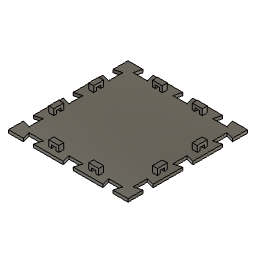
5 Power_source2 v14 (Autodesk Fusion 360 archive; units mm, degrees)
design "0 base_tile"
Autodesk Fusion 360 part; units mm, degrees
sketch "Sketch1" plane through (0, 0, 0) normal (0, 0, 1) x (1, 0, 0)
  line L0 (60, 60) -> (-60, 60)
  line L1 (-60, 60) -> (-60, -60)
  line L2 (-60, -60) -> (60, -60)
  line L3 (60, -60) -> (60, 60)
  line L4 (60, 60) -> (-60, -60) construction
  line L5 (-60, 60) -> (60, -60) construction
  dimension "d78" = 120
  dimension "d79" = 120
  constraint horizontal L0
  constraint perpendicular L0 L1
  constraint parallel L0 L2
  constraint parallel L1 L3
  constraint coincident L4 origin
  constraint coincident L5 origin
  measures "d78" distance of L1.end L2.end
  measures "d79" distance of L0.end L1.end
extrude "Extrude1" add sketch "Sketch1" along normal blind 3 makes body 1
sketch "Sketch3" plane through (0, 0, 3) normal (0, 0, 1) x (-1, 0, 0)
  line L0 (-60, 60) -> (-60, -60)
  line L1 (-60, -60) -> (60, -60)
  line L2 (60, -60) -> (60, 60)
  line L3 (60, 60) -> (-60, 60)
  line L4 (0, 60) -> (-5, 60)
  line L5 (0, 60) -> (5, 60)
  line L6 (5, 60) -> (7.0706, 52.2726)
  line L7 (5, 60) -> (13, 60) construction
  line L8 (-5, 60) -> (-7.0706, 52.2726)
  line L9 (-5, 60) -> (3, 60) construction
  line L10 (-7.0706, 52.2726) -> (7.0706, 52.2726)
  line L11 (-35, 60) -> (-32.9294, 52.2726)
  line L12 (-40, 60) -> (-35, 60)
  line L13 (-40, 60) -> (-45, 60)
  line L14 (-45, 60) -> (-47.0706, 52.2726)
  line L15 (-47.0706, 52.2726) -> (-32.9294, 52.2726)
  line L16 (45, 60) -> (47.0706, 52.2726)
  line L17 (40, 60) -> (45, 60)
  line L18 (40, 60) -> (35, 60)
  line L19 (35, 60) -> (32.9294, 52.2726)
  line L20 (32.9294, 52.2726) -> (47.0706, 52.2726)
  line L21 (-60, 45) -> (-52.2726, 47.0706)
  line L22 (-60, 40) -> (-60, 45)
  line L23 (-60, 40) -> (-60, 35)
  line L24 (-52.2726, 32.9294) -> (-52.2726, 47.0706)
  line L25 (-60, 35) -> (-52.2726, 32.9294)
  line L26 (-60, 5) -> (-52.2726, 7.0706)
  line L27 (-60, 0) -> (-60, 5)
  line L28 (-60, 0) -> (-60, -5)
  line L29 (-60, -5) -> (-52.2726, -7.0706)
  line L30 (-52.2726, -7.0706) -> (-52.2726, 7.0706)
  line L31 (-60, -35) -> (-52.2726, -32.9294)
  line L32 (-60, -40) -> (-60, -35)
  line L33 (-60, -40) -> (-60, -45)
  line L34 (-60, -45) -> (-52.2726, -47.0706)
  line L35 (-52.2726, -47.0706) -> (-52.2726, -32.9294)
  line L36 (-45, -60) -> (-47.0706, -52.2726)
  line L37 (-40, -60) -> (-45, -60)
  line L38 (-40, -60) -> (-35, -60)
  line L39 (-32.9294, -52.2726) -> (-47.0706, -52.2726)
  line L40 (-35, -60) -> (-32.9294, -52.2726)
  line L41 (-5, -60) -> (-7.0706, -52.2726)
  line L42 (0, -60) -> (-5, -60)
  line L43 (0, -60) -> (5, -60)
  line L44 (5, -60) -> (7.0706, -52.2726)
  line L45 (7.0706, -52.2726) -> (-7.0706, -52.2726)
  line L46 (35, -60) -> (32.9294, -52.2726)
  line L47 (40, -60) -> (35, -60)
  line L48 (40, -60) -> (45, -60)
  line L49 (45, -60) -> (47.0706, -52.2726)
  line L50 (47.0706, -52.2726) -> (32.9294, -52.2726)
  line L51 (60, -45) -> (52.2726, -47.0706)
  line L52 (60, -40) -> (60, -45)
  line L53 (60, -40) -> (60, -35)
  line L54 (52.2726, -32.9294) -> (52.2726, -47.0706)
  line L55 (60, -35) -> (52.2726, -32.9294)
  line L56 (60, -5) -> (52.2726, -7.0706)
  line L57 (60, 0) -> (60, -5)
  line L58 (60, 0) -> (60, 5)
  line L59 (60, 5) -> (52.2726, 7.0706)
  line L60 (52.2726, 7.0706) -> (52.2726, -7.0706)
  line L61 (60, 35) -> (52.2726, 32.9294)
  line L62 (60, 40) -> (60, 35)
  line L63 (60, 40) -> (60, 45)
  line L64 (60, 45) -> (52.2726, 47.0706)
  line L65 (52.2726, 47.0706) -> (52.2726, 32.9294)
  dimension "d92" = 5
  dimension "d93" = 5
  dimension "d94" = 75
  dimension "d95" = 8
  dimension "d96" = 105
  dimension "d97" = 8
  dimension "d100" = 40
  dimension "d101" = 0
  dimension "d103" = 360
  constraint midpoint L3 L4.start
  constraint parallel L3 L4
  constraint parallel L3 L5
  constraint horizontal L7
  constraint horizontal L9
  measures "d92" distance of L4.start L4.end
  measures "d93" distance of L4.start L5.end
  measures "d94" angle of L6 L7
  measures "d95" distance of L5.end L6.end
  measures "d96" angle of L8 L9
  measures "d97" distance of L4.end L8.end
extrude "Extrude4" cut sketch "Sketch3" against normal blind 3 contours L0 L21 L22 L23 L24 L25 | L3 L11 L12 L13 L14 L15 | L0 L26 L27 L28 L29 L30 | L3 L4 L5 L6 L8 L10 | L0 L31 L32 L33 L34 L35 | L3 L16 L17 L18 L19 L20 | L1 L36 L37 L38 L39 L40 | L2 L61 L62 L63 L64 L65 | L1 L41 L42 L43 L44 L45 | L2 L56 L57 L58 L59 L60 | L1 L46 L47 L48 L49 L50 | L2 L51 L52 L53 L54 L55 bodies 1
sketch "Sketch4" plane through (0, 0, 3) normal (0, 0, 1) x (-1, 0, 0)
  line L0 (-7.0706, 52.2726) -> (-5, 60)
  line L1 (-5, 60) -> (-35, 60)
  line L2 (-35, 60) -> (-32.9294, 52.2726)
  line L3 (-32.9294, 52.2726) -> (-47.0706, 52.2726)
  line L4 (-47.0706, 52.2726) -> (-45, 60)
  line L5 (-45, 60) -> (-60, 60)
  line L6 (-60, 60) -> (-60, 45)
  line L7 (-60, 45) -> (-52.2726, 47.0706)
  line L8 (-52.2726, 47.0706) -> (-52.2726, 32.9294)
  line L9 (-52.2726, 32.9294) -> (-60, 35)
  line L10 (-60, 35) -> (-60, 5)
  line L11 (-60, 5) -> (-52.2726, 7.0706)
  line L12 (-52.2726, 7.0706) -> (-52.2726, -7.0706)
  line L13 (-52.2726, -7.0706) -> (-60, -5)
  line L14 (-60, -5) -> (-60, -35)
  line L15 (-60, -35) -> (-52.2726, -32.9294)
  line L16 (-52.2726, -32.9294) -> (-52.2726, -47.0706)
  line L17 (-52.2726, -47.0706) -> (-60, -45)
  line L18 (-60, -45) -> (-60, -60)
  line L19 (-60, -60) -> (-45, -60)
  line L20 (-45, -60) -> (-47.0706, -52.2726)
  line L21 (-47.0706, -52.2726) -> (-32.9294, -52.2726)
  line L22 (-32.9294, -52.2726) -> (-35, -60)
  line L23 (-35, -60) -> (-5, -60)
  line L24 (-5, -60) -> (-7.0706, -52.2726)
  line L25 (-7.0706, -52.2726) -> (7.0706, -52.2726)
  line L26 (7.0706, -52.2726) -> (5, -60)
  line L27 (5, -60) -> (35, -60)
  line L28 (35, -60) -> (32.9294, -52.2726)
  line L29 (32.9294, -52.2726) -> (47.0706, -52.2726)
  line L30 (47.0706, -52.2726) -> (45, -60)
  line L31 (45, -60) -> (60, -60)
  line L32 (60, -60) -> (60, -45)
  line L33 (60, -45) -> (52.2726, -47.0706)
  line L34 (52.2726, -47.0706) -> (52.2726, -32.9294)
  line L35 (52.2726, -32.9294) -> (60, -35)
  line L36 (60, -35) -> (60, -5)
  line L37 (60, -5) -> (52.2726, -7.0706)
  line L38 (52.2726, -7.0706) -> (52.2726, 7.0706)
  line L39 (52.2726, 7.0706) -> (60, 5)
  line L40 (60, 5) -> (60, 35)
  line L41 (60, 35) -> (52.2726, 32.9294)
  line L42 (52.2726, 32.9294) -> (52.2726, 47.0706)
  line L43 (52.2726, 47.0706) -> (60, 45)
  line L44 (60, 45) -> (60, 60)
  line L45 (60, 60) -> (45, 60)
  line L46 (45, 60) -> (47.0706, 52.2726)
  line L47 (47.0706, 52.2726) -> (32.9294, 52.2726)
  line L48 (32.9294, 52.2726) -> (35, 60)
  line L49 (35, 60) -> (5, 60)
  line L50 (5, 60) -> (7.0706, 52.2726)
  line L51 (7.0706, 52.2726) -> (-7.0706, 52.2726)
  line L52 (0, 0) -> (0, 52) construction
  line L53 (0, 52) -> (20, 52) construction
  line L54 (15, 54.5) -> (25, 54.5)
  line L55 (25, 54.5) -> (25, 49.5)
  line L56 (25, 49.5) -> (15, 49.5)
  line L57 (15, 49.5) -> (15, 54.5)
  line L58 (15, 54.5) -> (25, 49.5) construction
  line L59 (25, 54.5) -> (15, 49.5) construction
  point P0 (20, 52)
  dimension "d106" = 52
  dimension "d107" = 20
  dimension "d108" = 10
  dimension "d109" = 5
  constraint coincident L52.start origin
  constraint perpendicular L51 L52
  constraint perpendicular L52 L53
  constraint horizontal L54
  constraint perpendicular L54 L55
  constraint parallel L54 L56
  constraint parallel L55 L57
  constraint coincident L58 P0
  constraint coincident L59 P0
  constraint coincident P0 L53.end
  measures "d106" distance of L52.start L52.end
  measures "d107" distance of L52.end P0
  measures "d108" distance of L55.end L56.end
  measures "d109" distance of L54.end L55.end
extrude "Extrude5" add sketch "Sketch4" along normal blind 6 separate body contours L54 L55 L56 L57 makes body 2
sketch "Sketch5" plane through (0, -54.5, 0) normal (0, -1, 0) x (1, 0, 0)
  line L0 (-15, 3) -> (-15, 9)
  line L1 (-15, 9) -> (-25, 9)
  line L2 (-25, 9) -> (-25, 3)
  line L3 (-20, 3) -> (-17.8, 3) construction
  line L4 (-17.8, 3) -> (-22.2, 3)
  line L5 (-22.2, 3) -> (-22.2, 6)
  line L6 (-22.2, 6) -> (-17.8, 6)
  line L7 (-17.8, 6) -> (-17.8, 3)
  line L8 (-25, 3) -> (-15, 3)
  dimension "d112" = 2.2
  dimension "d113" = 4.4
  dimension "d114" = 3
  constraint horizontal L4
  constraint vertical L5
  constraint horizontal L6
  constraint vertical L7
  measures "d112" distance of L3.start L3.end
  measures "d113" distance of L3.end L4.end
  measures "d114" distance of L3.end L6.end
extrude "zip_tie" cut sketch "Sketch5" against normal blind 5 contours L4 L5 L6 L7 L8 bodies 1 2
pattern_linear "R-Pattern1" count 2 spacing 40 along (1, 0, 0) of bodies 2 makes body 3
pattern_circular "C-Pattern1" count 4 over 360 about axis through (0, 0, 1.75) along (0, 0, 1) of bodies 2 3 makes body 4 at (52.8333, -18.3333, 9) makes body 5 at (21.6667, 51.1667, 9) makes body 6 at (-51.1667, 21.6667, 9) makes body 7 at (52.8333, 21.6667, 9) makes body 8 at (-18.3333, 52.8333, 9) makes body 9 at (-52.8333, -21.6667, 9)
sketch "Sketch6" plane through (0, 0, 0) normal (0, 1, 0) x (1, 0, 0)
equation "d108 = 4 mm + 3 mm + 3 mm"
equation "d110 = 3 mm + 3 mm"
named bodies: "tile", "zip_tie", "zip_tie (1)", "zip_tie (2)", "zip_tie (3)", "zip_tie (4)", "zip_tie (1) (1)", "zip_tie (1) (2)", "zip_tie (1) (3)"

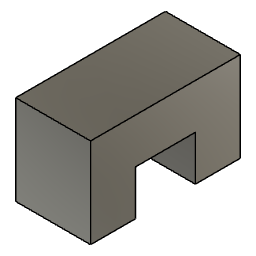
design "Zip_tie_holder"
Autodesk Fusion 360 part; units mm, degrees
sketch "Sketch1" plane through (0, 0, 0) normal (0, 0, 1) x (1, 0, 0)
  line L0 (-2.5, 5) -> (2.5, 5)
  line L1 (2.5, 5) -> (2.5, -5)
  line L2 (2.5, -5) -> (-2.5, -5)
  line L3 (-2.5, -5) -> (-2.5, 5)
  line L4 (-2.5, 5) -> (2.5, -5) construction
  line L5 (2.5, 5) -> (-2.5, -5) construction
  dimension "d1" = 5
  dimension "d2" = 10
  constraint horizontal L0
  constraint perpendicular L0 L1
  constraint parallel L0 L2
  constraint parallel L1 L3
  constraint coincident L4 origin
  constraint coincident L5 origin
  measures "d1" distance of L1.end L2.end
  measures "d2" distance of L0.end L1.end
extrude "Extrude1" add sketch "Sketch1" along normal blind 6
ref_plane "WorkPlane1" through (-2.5, 0, 3) normal (-1, 0, 0) x (0, -1, 0)
sketch "Sketch2" plane through (-2.5, 0, 0) normal (-1, 0, 0) x (0, -1, 0)
  line L0 (-2, 0) -> (2, 0)
  line L1 (2, 0) -> (2, 3)
  line L2 (2, 3) -> (-2, 3)
  line L3 (-2, 3) -> (-2, 0)
  dimension "d6" = 4
  dimension "d7" = 3
  constraint horizontal L0
  constraint vertical L1
  constraint horizontal L2
  constraint vertical L3
  measures "d6" distance of L0.start L0.end
  measures "d7" distance of L0.start L2.end
extrude "Extrude2" cut sketch "Sketch2" against normal blind 6
